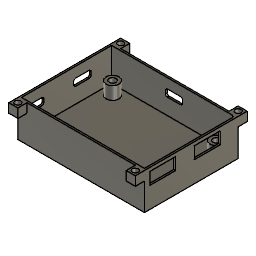
CASE bottom(f3d) (Autodesk Fusion 360 design; units mm, degrees)
part number: 2026-08-16-16-56-24-291
Autodesk Fusion 360 part; units mm, degrees
sketch "Sketch1" plane through (0, 0, 0) normal (0, 0, 1) x (1, 0, 0)
  line L0 (33.65, 24.65) -> (-33.65, 24.65)
  line L1 (-33.65, 24.65) -> (-33.65, -24.65)
  line L2 (-33.65, -24.65) -> (33.65, -24.65)
  line L3 (33.65, -24.65) -> (33.65, 24.65)
  line L4 (33.65, 24.65) -> (-33.65, -24.65) construction
  line L5 (-33.65, 24.65) -> (33.65, -24.65) construction
  line L6 (34.65, 25.65) -> (-34.65, 25.65)
  line L7 (-34.65, 25.65) -> (-34.65, -25.65)
  line L8 (-34.65, -25.65) -> (34.65, -25.65)
  line L9 (34.65, -25.65) -> (34.65, 25.65)
  line L10 (34.65, 25.65) -> (-34.65, -25.65) construction
  line L11 (-34.65, 25.65) -> (34.65, -25.65) construction
  line L12 (33.65, 24.65) -> (38.3726, 24.65)
  line L13 (38.3726, 24.65) -> (38.3726, 29.0356)
  line L14 (38.3726, 29.0356) -> (34.2811, 29.0356)
  line L15 (34.2811, 29.0356) -> (33.65, 24.65)
  line L16 (38.3726, 24.65) -> (34.2811, 29.0356) construction
  dimension "d1" = 67.3
  dimension "d2" = 49.3
  dimension "d3" = 69.3
  dimension "d4" = 51.3
  constraint horizontal L0
  constraint perpendicular L0 L1
  constraint parallel L0 L2
  constraint parallel L1 L3
  constraint coincident L4 origin
  constraint coincident L5 origin
  constraint horizontal L6
  constraint perpendicular L6 L7
  constraint parallel L6 L8
  constraint parallel L7 L9
  constraint coincident L10 origin
  constraint coincident L11 origin
  constraint horizontal L12
  constraint perpendicular L12 L13
  constraint parallel L12 L14
  measures "d1" distance of L1.end L2.end
  measures "d2" distance of L0.end L1.end
  measures "d3" distance of L7.end L8.end
  measures "d4" distance of L6.end L7.end
extrude "Extrude1" add sketch "Sketch1" along normal blind 2 contours L0 L1 L2 L3 makes body 1
extrude "Extrude2" add sketch "Sketch1" along normal blind 20 separate body contours L6 L9 L12 L15 | L6 L7 L8 L9 L12 L15 makes body 2
sketch "Sketch2" plane through (0, 0, 2) normal (0, 0, 1) x (-1, 0, 0)
  line L0 (-33.65, 24.65) -> (-33.65, -24.65)
  line L1 (-33.65, -24.65) -> (33.65, -24.65)
  line L2 (33.65, -24.65) -> (33.65, 24.65)
  line L3 (33.65, 24.65) -> (-33.65, 24.65)
  circle A0 centre (27.784, -19.31) radius 3.5
  circle A1 centre (-29.047, -19.31) radius 3.5
  line L4 (33.65, -24.65) -> (33.65, 24.65) construction
  line L5 (-33.65, -24.65) -> (33.65, -24.65) construction
  circle A2 centre (-0.835, 20.07) radius 3.5
  dimension "d9" = 7
  dimension "d10" = 7
  dimension "d11" = 5.866
  dimension "d12" = 5.34
  dimension "d14" = 5.34
  dimension "d15" = 7
  dimension "d16" = 34.485
  dimension "d20" = 4.603
  dimension "d21" = 4.58
  measures "d9" diameter of A0
  measures "d10" diameter of A1
  measures "d11" distance of A0.centre L4
  measures "d12" distance of A0.centre L5
  measures "d14" distance of A1.centre L5
  measures "d15" diameter of A2
  measures "d16" distance of L4 A2.centre
  measures "d20" distance of L0 A1.centre
  measures "d21" distance of L3 A2.centre
extrude "Extrude4" add sketch "Sketch2" along normal blind 7 contours A0 | A1 | A2 bodies 1
extrude "Extrude3" add sketch "Sketch2" along normal blind 3 contours A0 | A1 | A2 bodies 1
hole "Hole1" at (-27.784, 19.31, 9) direction (0, 0, -1) diameter 3.7 depth 6 tip angle 180 bodies 1
hole "Hole2" at (29.047, 19.31, 9) direction (0, 0, -1) diameter 3.7 depth 6 tip angle 180 bodies 1
hole "Hole3" at (0.835, -20.07, 9) direction (0, 0, -1) diameter 3.7 depth 6 tip angle 180 bodies 1
sketch "Sketch3" plane through (34.65, 0, 0) normal (1, 0, 0) x (0, 1, 0)
  line L0 (25.65, 0) -> (25.65, 20)
  line L1 (25.65, 20) -> (-25.65, 20)
  line L2 (-25.65, 20) -> (-25.65, 0)
  line L3 (-22.65, 18.064) -> (-8.65, 18.064)
  line L4 (-8.65, 18.064) -> (-8.65, 11.464)
  line L5 (-8.65, 11.464) -> (-22.65, 11.464)
  line L6 (-22.65, 11.464) -> (-22.65, 18.064)
  line L7 (1.65, 18.064) -> (15.85, 18.064)
  line L8 (15.85, 18.064) -> (15.85, 11.464)
  line L9 (15.85, 11.464) -> (1.65, 11.464)
  line L10 (1.65, 11.464) -> (1.65, 18.064)
  dimension "d33" = 14
  dimension "d34" = 6.6
  dimension "d35" = 14.2
  dimension "d36" = 6.6
  dimension "d37" = 3
  dimension "d38" = 9.8
  dimension "d39" = 1.936
  dimension "d40" = 1.936
  constraint horizontal L3
  constraint vertical L4
  constraint horizontal L5
  constraint vertical L6
  constraint horizontal L7
  constraint vertical L8
  constraint horizontal L9
  constraint vertical L10
  measures "d33" distance of L3.start L3.end
  measures "d34" distance of L3.start L5.end
  measures "d35" distance of L7.start L7.end
  measures "d36" distance of L7.start L9.end
  measures "d37" distance of L2 L6
  measures "d38" distance of L0 L8
  measures "d39" distance of L1 L3
  measures "d40" distance of L1 L7
extrude "Extrude5" cut sketch "Sketch3" against normal blind 2 bodies 2
sketch "Sketch4" plane through (0, 25.65, 0) normal (0, 1, 0) x (-1, 0, 0)
  line L0 (-34.65, 0) -> (34.65, 0)
  line L1 (34.65, 0) -> (34.65, 20)
  line L2 (34.65, 20) -> (-34.65, 20)
  line L3 (-34.65, 20) -> (-34.65, 0)
  line L4 (-5.15, 14.578) -> (4.15, 14.578)
  line L5 (4.15, 14.578) -> (4.15, 10.778)
  line L6 (4.15, 10.778) -> (-5.15, 10.778)
  line L7 (-5.15, 10.778) -> (-5.15, 14.578)
  dimension "d43" = 9.3
  dimension "d44" = 3.8
  dimension "d45" = 29.5
  dimension "d46" = 5.422
  constraint horizontal L4
  constraint vertical L5
  constraint horizontal L6
  constraint vertical L7
  measures "d43" distance of L4.start L4.end
  measures "d44" distance of L4.start L6.end
  measures "d45" distance of L3 L7
  measures "d46" distance of L2 L4
extrude "Extrude6" cut sketch "Sketch4" against normal blind 2 contours L4 L5 L6 L7 bodies 2
fillet "Fillet1" radius 1 4 edges at (-4.15, 25.15, 10.778) (-4.15, 25.15, 14.578) (5.15, 25.15, 14.578) (5.15, 25.15, 10.778) on bodies 2
sketch "Sketch5" plane through (-34.65, 0, 0) normal (-1, 0, 0) x (0, -1, 0)
  line L0 (-25.65, 0) -> (25.65, 0)
  line L1 (25.65, 0) -> (25.65, 20)
  line L2 (25.65, 20) -> (-25.65, 20)
  line L3 (-25.65, 20) -> (-25.65, 0)
  line L4 (-13.45, 14.3) -> (-3.95, 14.3)
  line L5 (-3.95, 14.3) -> (-3.95, 10.5)
  line L6 (-3.95, 10.5) -> (-13.45, 10.5)
  line L7 (-13.45, 10.5) -> (-13.45, 14.3)
  line L8 (12.41, 14.3) -> (21.91, 14.3)
  line L9 (21.91, 14.3) -> (21.91, 10.5)
  line L10 (21.91, 10.5) -> (12.41, 10.5)
  line L11 (12.41, 10.5) -> (12.41, 14.3)
  dimension "d51" = 9.5
  dimension "d52" = 3.8
  dimension "d53" = 9.5
  dimension "d54" = 3.8
  dimension "d55" = 12.2
  dimension "d56" = 3.74
  dimension "d57" = 5.7
  dimension "d58" = 5.7
  constraint horizontal L4
  constraint vertical L5
  constraint horizontal L6
  constraint vertical L7
  constraint horizontal L8
  constraint vertical L9
  constraint horizontal L10
  constraint vertical L11
  measures "d51" distance of L4.start L4.end
  measures "d52" distance of L4.start L6.end
  measures "d53" distance of L8.start L8.end
  measures "d54" distance of L8.start L10.end
  measures "d55" distance of L3 L7
  measures "d56" distance of L1 L9
  measures "d57" distance of L2 L8
  measures "d58" distance of L2 L4
extrude "Extrude7" cut sketch "Sketch5" against normal blind 2 contours L4 L5 L6 L7 bodies 2
extrude "Extrude8" cut sketch "Sketch5" against normal blind 2 contours L8 L9 L10 L11 bodies 2
fillet "Fillet2" radius 1 8 edges at (-34.15, 13.45, 14.3) (-34.15, 3.95, 14.3) (-34.15, 3.95, 10.5) (-34.15, 13.45, 10.5) (-34.15, -12.41, 10.5) (-34.15, -12.41, 14.3) (-34.15, -21.91, 14.3) (-34.15, -21.91, 10.5) on bodies 2
sketch "Sketch6" plane through (0, 25.65, 0) normal (0, 1, 0) x (-1, 0, 0)
  line L0 (4.15, 13.578) -> (4.15, 11.778)
  arc A0 (3.15, 10.778) -> (4.15, 11.778) centre (3.15, 11.778) ccw
  line L1 (3.15, 10.778) -> (-4.15, 10.778)
  arc A1 (-5.15, 11.778) -> (-4.15, 10.778) centre (-4.15, 11.778) ccw
  line L2 (-5.15, 11.778) -> (-5.15, 13.578)
  arc A2 (-4.15, 14.578) -> (-5.15, 13.578) centre (-4.15, 13.578) ccw
  line L3 (-4.15, 14.578) -> (3.15, 14.578)
  arc A3 (4.15, 13.578) -> (3.15, 14.578) centre (3.15, 13.578) ccw
  line L4 (-34.65, 0) -> (34.65, 0)
  line L5 (34.65, 0) -> (34.65, 20)
  line L6 (34.65, 20) -> (-34.65, 20)
  line L7 (-34.65, 20) -> (-34.65, 0)
fillet "Fillet3" radius 1 1 edges at (33.65, 24.65, 10) on bodies 2
sketch "Sketch11" plane through (0, 0, 20) normal (0, 0, 1) x (-1, 0, 0)
  line L0 (-33.65, -23.65) -> (-33.65, 24.65)
  line L1 (-33.65, 24.65) -> (33.65, 24.65)
  line L2 (33.65, 24.65) -> (33.65, -24.65)
  line L3 (33.65, -24.65) -> (-32.65, -24.65)
  arc A0 (-33.65, -23.65) -> (-32.65, -24.65) centre (-32.65, -23.65) ccw
  line L4 (-34.65, 25.65) -> (-34.65, -25.65)
  line L5 (-34.65, -25.65) -> (34.65, -25.65)
  line L6 (34.65, -25.65) -> (34.65, 25.65)
  line L7 (34.65, 25.65) -> (-34.65, 25.65)
  line L8 (34.65, -25.65) -> (29.65, -25.65)
  line L9 (29.65, -25.65) -> (29.65, -30.65)
  line L10 (29.65, -30.65) -> (34.65, -30.65)
  line L11 (34.65, -30.65) -> (34.65, -25.65)
  line L12 (-34.65, -25.65) -> (-29.65, -25.65)
  line L13 (-29.65, -25.65) -> (-29.65, -30.65)
  line L14 (-29.65, -30.65) -> (-34.65, -30.65)
  line L15 (-34.65, -30.65) -> (-34.65, -25.65)
  line L16 (-34.65, 25.65) -> (-29.65, 25.65)
  line L17 (-29.65, 25.65) -> (-29.65, 30.65)
  line L18 (-29.65, 30.65) -> (-34.65, 30.65)
  line L19 (-34.65, 30.65) -> (-34.65, 25.65)
  line L20 (34.65, 25.65) -> (29.65, 25.65)
  line L21 (29.65, 25.65) -> (29.65, 30.65)
  line L22 (29.65, 30.65) -> (34.65, 30.65)
  line L23 (34.65, 30.65) -> (34.65, 25.65)
  dimension "d110" = 5
  dimension "d111" = 5
  dimension "d112" = 5
  dimension "d113" = 5
  dimension "d114" = 5
  dimension "d115" = 5
  dimension "d116" = 5
  dimension "d117" = 5
  constraint horizontal L8
  constraint vertical L9
  constraint horizontal L10
  constraint vertical L11
  constraint coincident L5.end L6.start
  constraint horizontal L12
  constraint vertical L13
  constraint horizontal L14
  constraint vertical L15
  constraint coincident L4.end L5.start
  constraint horizontal L16
  constraint vertical L17
  constraint horizontal L18
  constraint vertical L19
  constraint coincident L4.start L7.end
  constraint horizontal L20
  constraint vertical L21
  constraint horizontal L22
  constraint vertical L23
  constraint coincident L6.end L7.start
  measures "d110" distance of L5.end L8.end
  measures "d111" distance of L5.end L10.end
  measures "d112" distance of L4.end L12.end
  measures "d113" distance of L4.end L14.end
  measures "d114" distance of L4.start L16.end
  measures "d115" distance of L4.start L18.end
  measures "d116" distance of L6.end L20.end
  measures "d117" distance of L6.end L22.end
extrude "Extrude12" add sketch "Sketch11" against normal blind 5 contours L7 L16 L17 L18 L19 | L5 L12 L13 L14 L15 | L7 L20 L21 L22 L23 | L5 L8 L9 L10 L11 bodies 2
sketch "Sketch12" plane through (0, 0, 20) normal (0, 0, 1) x (-1, 0, 0)
  line L0 (-33.65, -23.65) -> (-33.65, 24.65)
  line L1 (-33.65, 24.65) -> (33.65, 24.65)
  line L2 (33.65, 24.65) -> (33.65, -24.65)
  line L3 (33.65, -24.65) -> (-32.65, -24.65)
  arc A0 (-33.65, -23.65) -> (-32.65, -24.65) centre (-32.65, -23.65) ccw
  line L4 (-34.65, 30.65) -> (-34.65, -30.65)
  line L5 (-34.65, -30.65) -> (-29.65, -30.65)
  line L6 (-29.65, -30.65) -> (-29.65, -25.65)
  line L7 (-29.65, -25.65) -> (29.65, -25.65)
  line L8 (29.65, -25.65) -> (29.65, -30.65)
  line L9 (29.65, -30.65) -> (34.65, -30.65)
  line L10 (34.65, -30.65) -> (34.65, 30.65)
  line L11 (34.65, 30.65) -> (29.65, 30.65)
  line L12 (29.65, 30.65) -> (29.65, 25.65)
  line L13 (29.65, 25.65) -> (-29.65, 25.65)
  line L14 (-29.65, 25.65) -> (-29.65, 30.65)
  line L15 (-29.65, 30.65) -> (-34.65, 30.65)
  circle A1 centre (32.15, 28.15) radius 1.6
  circle A2 centre (32.15, -28.15) radius 1.6
  circle A3 centre (-32.15, -28.15) radius 1.6
  circle A4 centre (-32.15, 28.15) radius 1.6
  dimension "d120" = 3.2
  dimension "d121" = 3.2
  dimension "d122" = 3.2
  dimension "d123" = 3.2
  dimension "d124" = 2.5
  dimension "d125" = 2.5
  dimension "d126" = 2.5
  dimension "d127" = 2.5
  dimension "d128" = 2.5
  dimension "d129" = 2.5
  dimension "d130" = 2.5
  dimension "d131" = 2.5
  measures "d120" diameter of A1
  measures "d121" diameter of A2
  measures "d122" diameter of A3
  measures "d123" diameter of A4
  measures "d124" distance of L10 A2.centre
  measures "d125" distance of L9 A2.centre
  measures "d126" distance of L6 A3.centre
  measures "d127" distance of L5 A3.centre
  measures "d128" distance of L4 A4.centre
  measures "d129" distance of L15 A4.centre
  measures "d130" distance of L11 A1.centre
  measures "d131" distance of L10 A1.centre
extrude "Extrude13" cut sketch "Sketch12" against normal blind 3.1 contours A1 | A2 | A3 | A4 bodies 2
